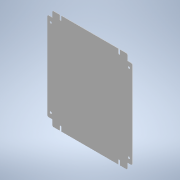
# Autodesk Inventor part: JBMP1614
Saved by Autodesk Inventor 2021 (Build 250183000, 183)
## iProperties
Created: 2025-08-10
Part Number: JBMP1614
Material: Generic
Catalog Web Link: www.cadenas.de
Description: Mounting plate JB-Small Enclosures
Vendor: RITTAL
Document SubType Name: Modeling
Designer: psAdmin
Manufacturer: RITTAL
Mass: 183.96 g
Surface Area: 2477.42 cm^2
Volume: 183.96 cm^3
Density: 1 g/cm^3
Appearance: PSOLRGB-175-175-175
Category: PARTsolutions
Company: RITTAL
Title: JBMP1614
Author: Cadenas PARTsolutions
Comments: Small Enclosures
PSOL_IDENT_0: {$CADENAS_DATA/23d-libs/rittal/schaltschranksys/kleingeh/jb_parts/jb_mounting_plate.prj},168 {VTYP=3
PSOL_IDENT_1: D},{NB=JBMP1614},{LINA=JBMP1614},{NN=Mounting plate JB},{DATE=28.09.2023 05:22:38},{GEOMDATE=28.09.2
PSOL_IDENT_2: 023 05:22:38},{VERSION=},{LINEID=100},{WBVAR=},{WBNUMERIC=}  {NB=JBMP1614},{LINA=JBMP1614},{KT=DUMMY
PSOL_IDENT_3: },{PN=JBMP1614},{BEST=8018198},{F1=325},{F2=50.0},{G1=385},{T1=1.500},{DETAIL=MIN}
NB: JBMP1614
NN: Mounting plate JB
NT: Small Enclosures
NBSYN: $PN.
LINA: JBMP1614
CATALOG: Rittal
PN: JBMP1614
BEST: 8018198
F1: 325
F2: 50
G1: 385
T1: 1.5
SUPPLIER: RITTAL
ARTICLENO: JBMP1614
BOMINFO: JBMP1614
CREATOR: CADENAS GmbH
Autodesk Inventor part; units mm, degrees
sketch "Sketch_1" plane through (0, 0, 0) normal (0, 0, 1) x (1, 0, 0)
  line L0 (-162.5, -166) -> (-159.5, -169)
  line L1 (-159.5, -169) -> (-144, -169)
  line L2 (-144, -169) -> (-144, -189.5)
  line L3 (-144, -189.5) -> (-141, -192.5)
  line L4 (-141, -192.5) -> (-116.1, -192.5)
  line L5 (-116.1, -192.5) -> (-116.1, -178)
  arc A0 (-108.9, -178) -> (-116.1, -178) centre (-112.5, -178) ccw
  line L6 (-108.9, -178) -> (-108.9, -192.5)
  line L7 (-108.9, -192.5) -> (108.9, -192.5)
  line L8 (108.9, -192.5) -> (108.9, -178)
  arc A1 (116.1, -178) -> (108.9, -178) centre (112.5, -178) ccw
  line L9 (116.1, -178) -> (116.1, -192.5)
  line L10 (116.1, -192.5) -> (141, -192.5)
  line L11 (141, -192.5) -> (144, -189.5)
  line L12 (144, -189.5) -> (144, -169)
  line L13 (144, -169) -> (159.5, -169)
  line L14 (159.5, -169) -> (162.5, -166)
  line L15 (162.5, -166) -> (162.5, 166)
  line L16 (162.5, 166) -> (159.5, 169)
  line L17 (159.5, 169) -> (144, 169)
  line L18 (144, 169) -> (144, 189.5)
  line L19 (144, 189.5) -> (141, 192.5)
  line L20 (141, 192.5) -> (116.1, 192.5)
  line L21 (116.1, 192.5) -> (116.1, 178)
  arc A2 (108.9, 178) -> (116.1, 178) centre (112.5, 178) ccw
  line L22 (108.9, 178) -> (108.9, 192.5)
  line L23 (108.9, 192.5) -> (-108.9, 192.5)
  line L24 (-108.9, 192.5) -> (-108.9, 178)
  arc A3 (-116.1, 178) -> (-108.9, 178) centre (-112.5, 178) ccw
  line L25 (-116.1, 178) -> (-116.1, 192.5)
  line L26 (-116.1, 192.5) -> (-141, 192.5)
  line L27 (-141, 192.5) -> (-144, 189.5)
  line L28 (-144, 189.5) -> (-144, 169)
  line L29 (-144, 169) -> (-159.5, 169)
  line L30 (-159.5, 169) -> (-162.5, 166)
  line L31 (-162.5, 166) -> (-162.5, -166)
  circle A4 centre (150, 150) radius 4.1
  circle A5 centre (150, -150) radius 4.1
  circle A6 centre (-150, 150) radius 4.1
  circle A7 centre (-150, -150) radius 4.1
  constraints: 64 end point, 8 centre point, 8 point on circle
extrude "Extrusion1" add sketch "Sketch_1" along normal blind 1.5
ref_plane "to_frame_XY" through (0, 0, 0) normal (0, 0, 1) x (1, 0, 0)
ref_plane "to_frame_YZ" through (0, 0, 0) normal (1, 0, 0) x (0, 1, 0)
ref_plane "to_frame_ZX" through (0, 0, 0) normal (0, 1, 0) x (0, 0, 1)
body "Solid1"
